Autodesk Inventor part; units mm, degrees
(part 5 of 7)
  line L3426 (-193.7386, -22.8386) -> (-193.9136, -22.7248)
  line L3427 (-193.9136, -22.7248) -> (-194.0733, -22.5914)
  line L3428 (-194.0733, -22.5914) -> (-194.216, -22.4401)
  line L3429 (-194.216, -22.4401) -> (-194.3401, -22.2722)
  line L3430 (-194.3401, -22.2722) -> (-194.4984, -22.0026)
  line L3431 (-194.4984, -22.0026) -> (-194.6175, -21.7136)
  line L3432 (-194.6175, -21.7136) -> (-194.7614, -21.1878)
  line L3433 (-194.7614, -21.1878) -> (-194.8323, -20.6472)
  line L3434 (-194.8323, -20.6472) -> (-194.8479, -20.2469)
  line L3435 (-194.8479, -20.2469) -> (-194.8362, -19.8464)
  line L3436 (-194.8323, 26.7434) -> (-194.7794, 27.1173)
  line L3437 (-194.7794, 27.1173) -> (-194.6772, 27.4752)
  line L3438 (-194.6772, 27.4752) -> (-194.5286, 27.8131)
  line L3439 (-194.5286, 27.8131) -> (-194.3367, 28.1265)
  line L3440 (-194.3367, 28.1265) -> (-194.1044, 28.4114)
  line L3441 (-194.1044, 28.4114) -> (-193.8348, 28.6634)
  line L3442 (-193.8348, 28.6634) -> (-193.5309, 28.8783)
  line L3443 (-193.5309, 28.8783) -> (-193.1956, 29.052)
  line L3444 (-193.1956, 29.052) -> (-192.8739, 29.1738)
  line L3445 (-192.8739, 29.1738) -> (-192.5434, 29.2669)
  line L3446 (-192.5434, 29.2669) -> (-192.2059, 29.3306)
  line L3447 (-192.2059, 29.3306) -> (-191.8636, 29.3645)
  line L3448 (-191.8636, 29.3645) -> (-191.5218, 29.3735)
  line L3449 (-191.5218, 29.3735) -> (-191.18, 29.3684)
  line L3450 (-191.18, 29.3684) -> (-191.18, 24.5364)
  line L3451 (-191.18, 24.5364) -> (-190.8858, 24.5593)
  line L3452 (-190.8858, 24.5593) -> (-190.5962, 24.6116)
  line L3453 (-190.5962, 24.6116) -> (-190.3134, 24.6926)
  line L3454 (-190.3134, 24.6926) -> (-190.0394, 24.802)
  line L3455 (-190.0394, 24.802) -> (-189.8038, 24.9316)
  line L3456 (-189.8038, 24.9316) -> (-189.5931, 25.0917)
  line L3457 (-189.5931, 25.0917) -> (-189.4096, 25.2786)
  line L3458 (-189.4096, 25.2786) -> (-189.2554, 25.489)
  line L3459 (-189.2554, 25.489) -> (-189.1329, 25.7192)
  line L3460 (-189.1329, 25.7192) -> (-189.0441, 25.9657)
  line L3461 (-189.0441, 25.9657) -> (-188.9913, 26.2249)
  line L3462 (-188.9913, 26.2249) -> (-188.9769, 26.4934)
  line L3463 (-188.9769, 26.4934) -> (-188.9951, 26.7775)
  line L3464 (-188.9951, 26.7775) -> (-189.055, 27.0559)
  line L3465 (-189.055, 27.0559) -> (-189.1523, 27.3014)
  line L3466 (-189.1523, 27.3014) -> (-189.2933, 27.5246)
  line L3467 (-189.2933, 27.5246) -> (-189.4825, 27.7331)
  line L3468 (-189.4825, 27.7331) -> (-189.7034, 27.9075)
  line L3469 (-189.7034, 27.9075) -> (-189.9949, 28.0747)
  line L3470 (-189.9949, 28.0747) -> (-190.305, 28.2043)
  line L3471 (-190.305, 28.2043) -> (-190.1644, 29.3411)
  line L3472 (-190.1644, 29.3411) -> (-189.8262, 29.2325)
  line L3473 (-189.8262, 29.2325) -> (-189.5048, 29.0844)
  line L3474 (-189.5048, 29.0844) -> (-189.2036, 28.8986)
  line L3475 (-189.2036, 28.8986) -> (-188.9261, 28.677)
  line L3476 (-188.9261, 28.677) -> (-188.6508, 28.3766)
  line L3477 (-188.6508, 28.3766) -> (-188.4271, 28.0391)
  line L3478 (-188.4271, 28.0391) -> (-188.2585, 27.6709)
  line L3479 (-188.2585, 27.6709) -> (-188.1487, 27.2786)
  line L3480 (-188.1487, 27.2786) -> (-188.0874, 26.8353)
  line L3481 (-188.0874, 26.8353) -> (-188.0749, 26.3893)
  line L3482 (-188.0749, 26.3893) -> (-188.111, 25.9446)
  line L3483 (-188.111, 25.9446) -> (-188.1956, 25.5051)
  line L3484 (-188.1956, 25.5051) -> (-188.3053, 25.1774)
  line L3485 (-188.3053, 25.1774) -> (-188.4537, 24.8698)
  line L3486 (-188.4537, 24.8698) -> (-188.6379, 24.5853)
  line L3487 (-188.6379, 24.5853) -> (-188.8553, 24.3267)
  line L3488 (-188.8553, 24.3267) -> (-189.103, 24.0971)
  line L3489 (-189.103, 24.0971) -> (-189.3783, 23.8992)
  line L3490 (-189.3783, 23.8992) -> (-189.6783, 23.7361)
  line L3491 (-189.6783, 23.7361) -> (-190.0003, 23.6106)
  line L3492 (-190.0003, 23.6106) -> (-190.3447, 23.5156)
  line L3493 (-190.3447, 23.5156) -> (-190.6949, 23.4486)
  line L3494 (-190.6949, 23.4486) -> (-191.0495, 23.4099)
  line L3495 (-191.0495, 23.4099) -> (-191.4065, 23.3996)
  line L3496 (-191.4065, 23.3996) -> (-191.7751, 23.4106)
  line L3497 (-191.7751, 23.4106) -> (-192.1412, 23.4495)
  line L3498 (-192.1412, 23.4495) -> (-192.5033, 23.5163)
  line L3499 (-192.5033, 23.5163) -> (-192.8597, 23.6106)
  line L3500 (-192.8597, 23.6106) -> (-193.1496, 23.7194)
  line L3501 (-193.1496, 23.7194) -> (-193.4237, 23.8577)
  line L3502 (-193.4237, 23.8577) -> (-193.6798, 24.0239)
  line L3503 (-193.6798, 24.0239) -> (-193.9159, 24.216)
  line L3504 (-193.9159, 24.216) -> (-194.1301, 24.4323)
  line L3505 (-194.1301, 24.4323) -> (-194.3205, 24.671)
  line L3506 (-194.3205, 24.671) -> (-194.4849, 24.9302)
  line L3507 (-194.4849, 24.9302) -> (-194.6214, 25.2082)
  line L3508 (-194.6214, 25.2082) -> (-194.7415, 25.5808)
  line L3509 (-194.7415, 25.5808) -> (-194.8171, 25.9634)
  line L3510 (-194.8171, 25.9634) -> (-194.8476, 26.3523)
  line L3511 (-194.8476, 26.3523) -> (-194.8323, 26.7434)
  line L3512 (-194.6995, -35.8152) -> (-194.6995, -34.7097)
  line L3513 (-194.6995, -34.7097) -> (-193.8479, -34.7097)
  line L3514 (-193.8479, -34.7097) -> (-193.8479, -35.8152)
  line L3515 (-193.8479, -35.8152) -> (-190.055, -35.8152)
  line L3516 (-190.055, -35.8152) -> (-189.7519, -35.8093)
  line L3517 (-189.7519, -35.8093) -> (-189.4534, -35.7566)
  line L3518 (-189.4534, -35.7566) -> (-189.3323, -35.6785)
  line L3519 (-189.3323, -35.6785) -> (-189.2386, -35.5691)
  line L3520 (-189.2386, -35.5691) -> (-189.1744, -35.3848)
  line L3521 (-189.1744, -35.3848) -> (-189.1604, -35.1902)
  line L3522 (-189.1604, -35.1902) -> (-189.1708, -34.949)
  line L3523 (-189.1708, -34.949) -> (-189.2034, -34.7097)
  line L3524 (-189.2034, -34.7097) -> (-188.2308, -34.5496)
  line L3525 (-188.2308, -34.5496) -> (-188.1681, -34.8873)
  line L3526 (-188.1681, -34.8873) -> (-188.1387, -35.2287)
  line L3527 (-188.1387, -35.2287) -> (-188.1426, -35.5714)
  line L3528 (-188.1426, -35.5714) -> (-188.18, -35.9128)
  line L3529 (-188.18, -35.9128) -> (-188.2439, -36.1415)
  line L3530 (-188.2439, -36.1415) -> (-188.3496, -36.3516)
  line L3531 (-188.3496, -36.3516) -> (-188.4935, -36.5377)
  line L3532 (-188.4935, -36.5377) -> (-188.6722, -36.6941)
  line L3533 (-188.6722, -36.6941) -> (-188.8197, -36.7661)
  line L3534 (-188.8197, -36.7661) -> (-188.9742, -36.8204)
  line L3535 (-188.9742, -36.8204) -> (-189.1338, -36.8564)
  line L3536 (-189.1338, -36.8564) -> (-189.2972, -36.8738)
  line L3537 (-189.2972, -36.8738) -> (-189.707, -36.8995)
  line L3538 (-189.707, -36.8995) -> (-190.1175, -36.9089)
  line L3539 (-190.1175, -36.9089) -> (-193.8479, -36.9089)
  line L3540 (-193.8479, -36.9089) -> (-193.8479, -37.7136)
  line L3541 (-193.8479, -37.7136) -> (-194.6995, -37.7136)
  line L3542 (-194.6995, -37.7136) -> (-194.6995, -36.9089)
  line L3543 (-194.6995, -36.9089) -> (-196.305, -36.9089)
  line L3544 (-196.305, -36.9089) -> (-196.9651, -35.8152)
  line L3545 (-196.9651, -35.8152) -> (-194.6995, -35.8152)
  line L3546 (-194.8401, 20.2825) -> (-194.8127, 20.5351)
  line L3547 (-194.8127, 20.5351) -> (-194.7541, 20.7814)
  line L3548 (-194.7541, 20.7814) -> (-194.6653, 21.0184)
  line L3549 (-194.6653, 21.0184) -> (-194.5472, 21.2434)
  line L3550 (-194.5472, 21.2434) -> (-194.3696, 21.4735)
  line L3551 (-194.3696, 21.4735) -> (-194.1547, 21.6657)
  line L3552 (-194.1547, 21.6657) -> (-193.9086, 21.8157)
  line L3553 (-193.9086, 21.8157) -> (-193.637, 21.9192)
  line L3554 (-193.637, 21.9192) -> (-193.3991, 21.9795)
  line L3555 (-193.3991, 21.9795) -> (-193.1576, 22.0212)
  line L3556 (-193.1576, 22.0212) -> (-192.9136, 22.0441)
  line L3557 (-192.9136, 22.0441) -> (-192.6683, 22.0481)
  line L3558 (-192.6683, 22.0481) -> (-188.219, 22.0481)
  line L3559 (-188.219, 22.0481) -> (-188.219, 20.9583)
  line L3560 (-188.219, 20.9583) -> (-192.3011, 20.9583)
  line L3561 (-192.3011, 20.9583) -> (-192.6934, 20.9484)
  line L3562 (-192.6934, 20.9484) -> (-193.0823, 20.8958)
  line L3563 (-193.0823, 20.8958) -> (-193.274, 20.8411)
  line L3564 (-193.274, 20.8411) -> (-193.4477, 20.748)
  line L3565 (-193.4477, 20.748) -> (-193.598, 20.6205)
  line L3566 (-193.598, 20.6205) -> (-193.719, 20.4622)
  line L3567 (-193.719, 20.4622) -> (-193.8114, 20.2685)
  line L3568 (-193.8114, 20.2685) -> (-193.8707, 20.0638)
  line L3569 (-193.8707, 20.0638) -> (-193.8962, 19.8523)
  line L3570 (-193.8962, 19.8523) -> (-193.887, 19.6379)
  line L3571 (-193.887, 19.6379) -> (-193.8564, 19.4131)
  line L3572 (-193.8564, 19.4131) -> (-193.7925, 19.1996)
  line L3573 (-193.7925, 19.1996) -> (-193.6978, 19.0006)
  line L3574 (-193.6978, 19.0006) -> (-193.5748, 18.819)
  line L3575 (-193.5748, 18.819) -> (-193.4259, 18.658)
  line L3576 (-193.4259, 18.658) -> (-193.2534, 18.5207)
  line L3577 (-193.2534, 18.5207) -> (-193.06, 18.4101)
  line L3578 (-193.06, 18.4101) -> (-192.8479, 18.3293)
  line L3579 (-192.8479, 18.3293) -> (-192.4207, 18.2395)
  line L3580 (-192.4207, 18.2395) -> (-191.9847, 18.2161)
  line L3581 (-191.9847, 18.2161) -> (-188.219, 18.2161)
  line L3582 (-188.219, 18.2161) -> (-188.219, 17.1184)
  line L3583 (-188.219, 17.1184) -> (-192.43, 17.1184)
  line L3584 (-192.43, 17.1184) -> (-192.7524, 17.1051)
  line L3585 (-192.7524, 17.1051) -> (-193.0706, 17.052)
  line L3586 (-193.0706, 17.052) -> (-193.3245, 16.9661)
  line L3587 (-193.3245, 16.9661) -> (-193.5276, 16.8489)
  line L3588 (-193.5276, 16.8489) -> (-193.658, 16.7293)
  line L3589 (-193.658, 16.7293) -> (-193.7605, 16.5873)
  line L3590 (-193.7605, 16.5873) -> (-193.8326, 16.4277)
  line L3591 (-193.8326, 16.4277) -> (-193.8714, 16.2551)
  line L3592 (-193.8714, 16.2551) -> (-193.8959, 15.9585)
  line L3593 (-193.8959, 15.9585) -> (-193.8667, 15.6647)
  line L3594 (-193.8667, 15.6647) -> (-193.7851, 15.381)
  line L3595 (-193.7851, 15.381) -> (-193.6526, 15.1145)
  line L3596 (-193.6526, 15.1145) -> (-193.5526, 14.9735)
  line L3597 (-193.5526, 14.9735) -> (-193.4355, 14.8474)
  line L3598 (-193.4355, 14.8474) -> (-193.3029, 14.7376)
  line L3599 (-193.3029, 14.7376) -> (-193.1565, 14.6458)
  line L3600 (-193.1565, 14.6458) -> (-192.9228, 14.5385)
  line L3601 (-192.9228, 14.5385) -> (-192.6761, 14.4661)
  line L3602 (-192.6761, 14.4661) -> (-192.1319, 14.3864)
  line L3603 (-192.1319, 14.3864) -> (-191.5823, 14.3645)
  line L3604 (-191.5823, 14.3645) -> (-188.219, 14.3645)
  line L3605 (-188.219, 14.3645) -> (-188.219, 13.2668)
  line L3606 (-188.219, 13.2668) -> (-194.6995, 13.2668)
  line L3607 (-194.6995, 13.2668) -> (-194.6995, 14.2512)
  line L3608 (-194.6995, 14.2512) -> (-193.7933, 14.2512)
  line L3609 (-193.7933, 14.2512) -> (-194.0001, 14.3989)
  line L3610 (-194.0001, 14.3989) -> (-194.1874, 14.5672)
  line L3611 (-194.1874, 14.5672) -> (-194.3537, 14.7542)
  line L3612 (-194.3537, 14.7542) -> (-194.498, 14.9579)
  line L3613 (-194.498, 14.9579) -> (-194.6188, 15.1763)
  line L3614 (-194.6188, 15.1763) -> (-194.715, 15.4074)
  line L3615 (-194.715, 15.4074) -> (-194.7853, 15.6492)
  line L3616 (-194.7853, 15.6492) -> (-194.8284, 15.8997)
  line L3617 (-194.8284, 15.8997) -> (-194.8467, 16.143)
  line L3618 (-194.8467, 16.143) -> (-194.8436, 16.3864)
  line L3619 (-194.8436, 16.3864) -> (-194.8193, 16.6287)
  line L3620 (-194.8193, 16.6287) -> (-194.7737, 16.8684)
  line L3621 (-194.7737, 16.8684) -> (-194.68, 17.1497)
  line L3622 (-194.68, 17.1497) -> (-194.588, 17.3313)
  line L3623 (-194.588, 17.3313) -> (-194.4751, 17.4999)
  line L3624 (-194.4751, 17.4999) -> (-194.3425, 17.6534)
  line L3625 (-194.3425, 17.6534) -> (-194.1917, 17.7903)
  line L3626 (-194.1917, 17.7903) -> (-193.9617, 17.9366)
  line L3627 (-193.9617, 17.9366) -> (-193.7112, 18.0442)
  line L3628 (-193.7112, 18.0442) -> (-193.9614, 18.2279)
  line L3629 (-193.9614, 18.2279) -> (-194.1882, 18.4384)
  line L3630 (-194.1882, 18.4384) -> (-194.3894, 18.6735)
  line L3631 (-194.3894, 18.6735) -> (-194.5628, 18.9309)
  line L3632 (-194.5628, 18.9309) -> (-194.6614, 19.1236)
  line L3633 (-194.6614, 19.1236) -> (-194.739, 19.325)
  line L3634 (-194.739, 19.325) -> (-194.7948, 19.5335)
  line L3635 (-194.7948, 19.5335) -> (-194.8284, 19.7473)
  line L3636 (-194.8284, 19.7473) -> (-194.8474, 20.0146)
  line L3637 (-194.8474, 20.0146) -> (-194.8401, 20.2825)
  line L3638 (-188.219, 11.6223) -> (-188.219, 10.5247)
  line L3639 (-188.219, 10.5247) -> (-194.6995, 10.5247)
  line L3640 (-194.6995, 10.5247) -> (-194.6995, 11.6223)
  line L3641 (-194.6995, 11.6223) -> (-188.219, 11.6223)
  line L3642 (-197.1644, -2.0066) -> (-197.1365, -1.3334)
  line L3643 (-197.1365, -1.3334) -> (-197.0394, -0.6667)
  line L3644 (-197.0394, -0.6667) -> (-196.9661, -0.397)
  line L3645 (-196.9661, -0.397) -> (-196.8703, -0.1349)
  line L3646 (-196.8703, -0.1349) -> (-196.7526, 0.1181)
  line L3647 (-196.7526, 0.1181) -> (-196.6136, 0.3606)
  line L3648 (-196.6136, 0.3606) -> (-196.3987, 0.6458)
  line L3649 (-196.3987, 0.6458) -> (-196.0784, 0.9778)
  line L3650 (-196.0784, 0.9778) -> (-195.7151, 1.2629)
  line L3651 (-195.7151, 1.2629) -> (-195.3128, 1.5051)
  line L3652 (-195.3128, 1.5051) -> (-194.8675, 1.7043)
  line L3653 (-194.8675, 1.7043) -> (-194.387, 1.8567)
  line L3654 (-194.387, 1.8567) -> (-193.8596, 1.968)
  line L3655 (-193.8596, 1.968) -> (-193.3245, 2.0325)
  line L3656 (-193.3245, 2.0325) -> (-192.9384, 2.0538)
  line L3657 (-192.9384, 2.0538) -> (-192.552, 2.0544)
  line L3658 (-192.552, 2.0544) -> (-192.1661, 2.0342)
  line L3659 (-192.1661, 2.0342) -> (-191.7815, 1.9934)
  line L3660 (-191.7815, 1.9934) -> (-191.2923, 1.9097)
  line L3661 (-191.2923, 1.9097) -> (-190.8145, 1.7795)
  line L3662 (-190.8145, 1.7795) -> (-190.3515, 1.6039)
  line L3663 (-190.3515, 1.6039) -> (-189.9065, 1.384)
  line L3664 (-189.9065, 1.384) -> (-189.5949, 1.1825)
  line L3665 (-189.5949, 1.1825) -> (-189.3083, 0.9484)
  line L3666 (-189.3083, 0.9484) -> (-189.0494, 0.6841)
  line L3667 (-189.0494, 0.6841) -> (-188.8206, 0.3918)
  line L3668 (-188.8206, 0.3918) -> (-188.6377, 0.0648)
  line L3669 (-188.6377, 0.0648) -> (-188.4901, -0.2785)
  line L3670 (-188.4901, -0.2785) -> (-188.3788, -0.6353)
  line L3671 (-188.3788, -0.6353) -> (-188.305, -1.0027)
  line L3672 (-188.305, -1.0027) -> (-188.2376, -1.5574)
  line L3673 (-188.2376, -1.5574) -> (-188.219, -2.116)
  line L3674 (-188.219, -2.116) -> (-188.219, -5.3425)
  line L3675 (-188.219, -5.3425) -> (-197.1683, -5.3425)
  line L3676 (-197.1683, -5.3425) -> (-197.1683, -2.2605)
  line L3677 (-197.1683, -2.2605) -> (-197.1644, -2.0066)
  line L3678 (-194.8362, -12.6433) -> (-194.7875, -12.3186)
  line L3679 (-194.7875, -12.3186) -> (-194.6967, -12.0045)
  line L3680 (-194.6967, -12.0045) -> (-194.5653, -11.7052)
  line L3681 (-194.5653, -11.7052) -> (-194.3948, -11.4246)
  line L3682 (-194.3948, -11.4246) -> (-194.2515, -11.2623)
  line L3683 (-194.2515, -11.2623) -> (-194.0882, -11.1217)
  line L3684 (-194.0882, -11.1217) -> (-193.9073, -11.0046)
  line L3685 (-193.9073, -11.0046) -> (-193.7112, -10.9128)
  line L3686 (-193.7112, -10.9128) -> (-193.504, -10.8357)
  line L3687 (-193.504, -10.8357) -> (-193.2906, -10.7799)
  line L3688 (-193.2906, -10.7799) -> (-193.0726, -10.7456)
  line L3689 (-193.0726, -10.7456) -> (-192.8519, -10.7332)
  line L3690 (-192.8519, -10.7332) -> (-192.5278, -10.7206)
  line L3691 (-192.5278, -10.7206) -> (-192.2034, -10.7175)
  line L3692 (-192.2034, -10.7175) -> (-188.219, -10.7175)
  line L3693 (-188.219, -10.7175) -> (-188.219, -11.8152)
  line L3694 (-188.219, -11.8152) -> (-192.1604, -11.8152)
  line L3695 (-192.1604, -11.8152) -> (-192.5707, -11.8269)
  line L3696 (-192.5707, -11.8269) -> (-192.9769, -11.8855)
  line L3697 (-192.9769, -11.8855) -> (-193.2395, -11.9747)
  line L3698 (-193.2395, -11.9747) -> (-193.4685, -12.124)
  line L3699 (-193.4685, -12.124) -> (-193.6538, -12.3249)
  line L3700 (-193.6538, -12.3249) -> (-193.7854, -12.5691)
  line L3701 (-193.7854, -12.5691) -> (-193.8689, -12.8607)
  line L3702 (-193.8689, -12.8607) -> (-193.8948, -13.1628)
  line L3703 (-193.8948, -13.1628) -> (-193.8675, -13.5027)
  line L3704 (-193.8675, -13.5027) -> (-193.7854, -13.8191)
  line L3705 (-193.7854, -13.8191) -> (-193.6448, -14.1082)
  line L3706 (-193.6448, -14.1082) -> (-193.4495, -14.3738)
  line L3707 (-193.4495, -14.3738) -> (-193.3097, -14.5026)
  line L3708 (-193.3097, -14.5026) -> (-193.1541, -14.6103)
  line L3709 (-193.1541, -14.6103) -> (-192.9851, -14.6955)
  line L3710 (-192.9851, -14.6955) -> (-192.805, -14.7566)
  line L3711 (-192.805, -14.7566) -> (-192.5474, -14.8178)
  line L3712 (-192.5474, -14.8178) -> (-192.2863, -14.8598)
  line L3713 (-192.2863, -14.8598) -> (-192.0229, -14.8824)
  line L3714 (-192.0229, -14.8824) -> (-191.7581, -14.8855)
  line L3715 (-191.7581, -14.8855) -> (-188.219, -14.8855)
  line L3716 (-188.219, -14.8855) -> (-188.219, -15.9832)
  line L3717 (-188.219, -15.9832) -> (-194.6995, -15.9832)
  line L3718 (-194.6995, -15.9832) -> (-194.6995, -14.9949)
  line L3719 (-194.6995, -14.9949) -> (-193.7776, -14.9949)
  line L3720 (-193.7776, -14.9949) -> (-194.0195, -14.816)
  line L3721 (-194.0195, -14.816) -> (-194.2358, -14.6087)
  line L3722 (-194.2358, -14.6087) -> (-194.4242, -14.3758)
  line L3723 (-194.4242, -14.3758) -> (-194.5823, -14.1199)
  line L3724 (-194.5823, -14.1199) -> (-194.702, -13.8366)
  line L3725 (-194.702, -13.8366) -> (-194.7866, -13.5421)
  line L3726 (-194.7866, -13.5421) -> (-194.8355, -13.2396)
  line L3727 (-194.8355, -13.2396) -> (-194.8479, -12.9324)
  line L3728 (-194.8479, -12.9324) -> (-194.8362, -12.6433)
  line L3729 (-197.3128, -24.3152) -> (-197.2749, -23.919)
  line L3730 (-197.2749, -23.919) -> (-197.2112, -23.5261)
  line L3731 (-197.2112, -23.5261) -> (-196.2503, -23.6902)
  line L3732 (-196.2503, -23.6902) -> (-196.2963, -24.013)
  line L3733 (-196.2963, -24.013) -> (-196.3128, -24.3386)
  line L3734 (-196.3128, -24.3386) -> (-196.2993, -24.5533)
  line L3735 (-196.2993, -24.5533) -> (-196.2581, -24.7644)
  line L3736 (-196.2581, -24.7644) -> (-196.1968, -24.9157)
  line L3737 (-196.1968, -24.9157) -> (-196.0979, -25.0457)
  line L3738 (-196.0979, -25.0457) -> (-195.969, -25.1355)
  line L3739 (-195.969, -25.1355) -> (-195.7748, -25.207)
  line L3740 (-195.7748, -25.207) -> (-195.5706, -25.241)
  line L3741 (-195.5706, -25.241) -> (-195.1352, -25.2563)
  line L3742 (-195.1352, -25.2563) -> (-194.6995, -25.2527)
  line L3743 (-194.6995, -25.2527) -> (-194.6995, -23.991)
  line L3744 (-194.6995, -23.991) -> (-193.8479, -23.991)
  line L3745 (-193.8479, -23.991) -> (-193.8479, -25.2527)
  line L3746 (-193.8479, -25.2527) -> (-188.219, -25.2527)
  line L3747 (-188.219, -25.2527) -> (-188.219, -26.3464)
  line L3748 (-188.219, -26.3464) -> (-193.8479, -26.3464)
  line L3749 (-193.8479, -26.3464) -> (-193.8479, -27.3152)
  line L3750 (-193.8479, -27.3152) -> (-194.6995, -27.3152)
  line L3751 (-194.6995, -27.3152) -> (-194.6995, -26.3464)
  line L3752 (-194.6995, -26.3464) -> (-195.1976, -26.3489)
  line L3753 (-195.1976, -26.3489) -> (-195.6956, -26.3386)
  line L3754 (-195.6956, -26.3386) -> (-196.0317, -26.3088)
  line L3755 (-196.0317, -26.3088) -> (-196.3597, -26.2293)
  line L3756 (-196.3597, -26.2293) -> (-196.6195, -26.1015)
  line L3757 (-196.6195, -26.1015) -> (-196.8453, -25.9252)
  line L3758 (-196.8453, -25.9252) -> (-197.0304, -25.7065)
  line L3759 (-197.0304, -25.7065) -> (-197.1683, -25.4519)
  line L3760 (-197.1683, -25.4519) -> (-197.2542, -25.1902)
  line L3761 (-197.2542, -25.1902) -> (-197.3134, -24.7547)
  line L3762 (-197.3134, -24.7547) -> (-197.3128, -24.3152)
  line L3763 (-188.219, 31.8411) -> (-188.219, 30.7434)
  line L3764 (-188.219, 30.7434) -> (-197.1683, 30.7434)
  line L3765 (-197.1683, 30.7434) -> (-197.1683, 31.8411)
  line L3766 (-197.1683, 31.8411) -> (-188.219, 31.8411)
  line L3767 (-191.4104, -19.0027) -> (-191.1986, -19.8133)
  line L3768 (-191.1986, -19.8133) -> (-191.0589, -20.6394)
  line L3769 (-191.0589, -20.6394) -> (-190.9765, -21.1247)
  line L3770 (-190.9765, -21.1247) -> (-190.8362, -21.5964)
  line L3771 (-190.8362, -21.5964) -> (-190.6926, -21.84)
  line L3772 (-190.6926, -21.84) -> (-190.4877, -22.0259)
  line L3773 (-190.4877, -22.0259) -> (-190.2373, -22.1435)
  line L3774 (-190.2373, -22.1435) -> (-189.9573, -22.1824)
  line L3775 (-189.9573, -22.1824) -> (-189.7515, -22.1639)
  line L3776 (-189.7515, -22.1639) -> (-189.555, -22.1003)
  line L3777 (-189.555, -22.1003) -> (-189.4166, -22.0194)
  line L3778 (-189.4166, -22.0194) -> (-189.2929, -21.9189)
  line L3779 (-189.2929, -21.9189) -> (-189.186, -21.8007)
  line L3780 (-189.186, -21.8007) -> (-189.0979, -21.6668)
  line L3781 (-189.0979, -21.6668) -> (-189.0047, -21.4288)
  line L3782 (-189.0047, -21.4288) -> (-188.9534, -21.1785)
  line L3783 (-188.9534, -21.1785) -> (-188.9323, -20.8798)
  line L3784 (-188.9323, -20.8798) -> (-188.9483, -20.582)
  line L3785 (-188.9483, -20.582) -> (-189.0011, -20.2885)
  line L3786 (-189.0011, -20.2885) -> (-189.0901, -20.0027)
  line L3787 (-189.0901, -20.0027) -> (-189.1751, -19.8148)
  line L3788 (-189.1751, -19.8148) -> (-189.2789, -19.6374)
  line L3789 (-189.2789, -19.6374) -> (-189.4007, -19.4716)
  line L3790 (-189.4007, -19.4716) -> (-189.5394, -19.3191)
  line L3791 (-189.5394, -19.3191) -> (-189.7431, -19.1546)
  line L3792 (-189.7431, -19.1546) -> (-189.969, -19.0222)
  line L3793 (-189.969, -19.0222) -> (-190.3406, -18.9061)
  line L3794 (-190.3406, -18.9061) -> (-190.7269, -18.8582)
  line L3795 (-190.7269, -18.8582) -> (-191.0998, -18.8459)
  line L3796 (-191.0998, -18.8459) -> (-191.4729, -18.8464)
  line L3797 (-191.4729, -18.8464) -> (-191.4104, -19.0027)
  line L3798 (-196.1097, -4.1589) -> (-189.2737, -4.1589)
  line L3799 (-189.2737, -4.1589) -> (-189.2737, -2.2488)
  line L3800 (-189.2737, -2.2488) -> (-189.293, -1.6898)
  line L3801 (-189.293, -1.6898) -> (-189.3675, -1.1355)
  line L3802 (-189.3675, -1.1355) -> (-189.4284, -0.8919)
  line L3803 (-189.4284, -0.8919) -> (-189.515, -0.657)
  line L3804 (-189.515, -0.657) -> (-189.6265, -0.4328)
  line L3805 (-189.6265, -0.4328) -> (-189.762, -0.2214)
  line L3806 (-189.762, -0.2214) -> (-189.9026, -0.0574)
  line L3807 (-189.9026, -0.0574) -> (-190.0834, 0.101)
  line L3808 (-190.0834, 0.101) -> (-190.2773, 0.2422)
  line L3809 (-190.2773, 0.2422) -> (-190.483, 0.3655)
  line L3810 (-190.483, 0.3655) -> (-190.6995, 0.47)
  line L3811 (-190.6995, 0.47) -> (-190.9715, 0.5747)
  line L3812 (-190.9715, 0.5747) -> (-191.2496, 0.6606)
  line L3813 (-191.2496, 0.6606) -> (-191.533, 0.7273)
  line L3814 (-191.533, 0.7273) -> (-191.8206, 0.7747)
  line L3815 (-191.8206, 0.7747) -> (-192.2955, 0.8194)
  line L3816 (-192.2955, 0.8194) -> (-192.7719, 0.8336)
  line L3817 (-192.7719, 0.8336) -> (-193.2482, 0.8174)
  line L3818 (-193.2482, 0.8174) -> (-193.7229, 0.7708)
  line L3819 (-193.7229, 0.7708) -> (-193.9794, 0.726)
  line L3820 (-193.9794, 0.726) -> (-194.2316, 0.6627)
  line L3821 (-194.2316, 0.6627) -> (-194.4785, 0.5812)
  line L3822 (-194.4785, 0.5812) -> (-194.719, 0.4817)
  line L3823 (-194.719, 0.4817) -> (-195.0263, 0.3093)
  line L3824 (-195.0263, 0.3093) -> (-195.3063, 0.0981)
  line L3825 (-195.3063, 0.0981) -> (-195.5554, -0.1489)
  line L3826 (-195.5554, -0.1489) -> (-195.7698, -0.4285)
  line L3827 (-195.7698, -0.4285) -> (-195.8835, -0.6501)
  line L3828 (-195.8835, -0.6501) -> (-195.9713, -0.8824)
  line L3829 (-195.9713, -0.8824) -> (-196.0326, -1.1231)
  line L3830 (-196.0326, -1.1231) -> (-196.0667, -1.3699)
  line L3831 (-196.0667, -1.3699) -> (-196.0928, -1.6957)
  line L3832 (-196.0928, -1.6957) -> (-196.1097, -2.0222)
  line L3833 (-196.1097, -2.0222) -> (-196.1097, -4.1589)
  line L3834 (-193.9378, 6.0051) -> (-193.8934, 5.7383)
  line L3835 (-193.8934, 5.7383) -> (-193.811, 5.4854)
  line L3836 (-193.811, 5.4854) -> (-193.6932, 5.2501)
  line L3837 (-193.6932, 5.2501) -> (-193.543, 5.0355)
  line L3838 (-193.543, 5.0355) -> (-193.3629, 4.8453)
  line L3839 (-193.3629, 4.8453) -> (-193.1559, 4.6827)
  line L3840 (-193.1559, 4.6827) -> (-192.9247, 4.5513)
  line L3841 (-192.9247, 4.5513) -> (-192.6722, 4.4543)
  line L3842 (-192.6722, 4.4543) -> (-192.3803, 4.3834)
  line L3843 (-192.3803, 4.3834) -> (-192.0823, 4.345)
  line L3844 (-192.0823, 4.345) -> (-192.0823, 7.9661)
  line L3845 (-192.0823, 7.9661) -> (-192.4436, 7.9157)
  line L3846 (-192.4436, 7.9157) -> (-192.7972, 7.8254)
  line L3847 (-192.7972, 7.8254) -> (-193.0784, 7.7043)
  line L3848 (-193.0784, 7.7043) -> (-193.3089, 7.552)
  line L3849 (-193.3089, 7.552) -> (-193.5836, 7.2736)
  line L3850 (-193.5836, 7.2736) -> (-193.7856, 6.9443)
  line L3851 (-193.7856, 6.9443) -> (-193.9085, 6.5781)
  line L3852 (-193.9085, 6.5781) -> (-193.9456, 6.1887)
  line L3853 (-193.9456, 6.1887) -> (-193.9378, 6.0051)
  line L3854 (-193.9378, -31.1199) -> (-193.8934, -31.3867)
  line L3855 (-193.8934, -31.3867) -> (-193.811, -31.6396)
  line L3856 (-193.811, -31.6396) -> (-193.6932, -31.8749)
  line L3857 (-193.6932, -31.8749) -> (-193.543, -32.0895)
  line L3858 (-193.543, -32.0895) -> (-193.3629, -32.2797)
  line L3859 (-193.3629, -32.2797) -> (-193.1559, -32.4423)
  line L3860 (-193.1559, -32.4423) -> (-192.9247, -32.5737)
  line L3861 (-192.9247, -32.5737) -> (-192.6722, -32.6707)
  line L3862 (-192.6722, -32.6707) -> (-192.3803, -32.7416)
  line L3863 (-192.3803, -32.7416) -> (-192.0823, -32.78)
  line L3864 (-192.0823, -32.78) -> (-192.0823, -29.1589)
  line L3865 (-192.0823, -29.1589) -> (-192.4436, -29.2093)
  line L3866 (-192.4436, -29.2093) -> (-192.7972, -29.2996)
  line L3867 (-192.7972, -29.2996) -> (-193.0784, -29.4207)
  line L3868 (-193.0784, -29.4207) -> (-193.3089, -29.573)
  line L3869 (-193.3089, -29.573) -> (-193.5836, -29.8514)
  line L3870 (-193.5836, -29.8514) -> (-193.7856, -30.1807)
  line L3871 (-193.7856, -30.1807) -> (-193.9085, -30.5469)
  line L3872 (-193.9085, -30.5469) -> (-193.9456, -30.9363)
  line L3873 (-193.9456, -30.9363) -> (-193.9378, -31.1199)
  line L3874 (-193.9378, 26.2551) -> (-193.8934, 25.9883)
  line L3875 (-193.8934, 25.9883) -> (-193.811, 25.7354)
  line L3876 (-193.811, 25.7354) -> (-193.6932, 25.5001)
  line L3877 (-193.6932, 25.5001) -> (-193.543, 25.2855)
  line L3878 (-193.543, 25.2855) -> (-193.3629, 25.0953)
  line L3879 (-193.3629, 25.0953) -> (-193.1559, 24.9327)
  line L3880 (-193.1559, 24.9327) -> (-192.9247, 24.8013)
  line L3881 (-192.9247, 24.8013) -> (-192.6722, 24.7043)
  line L3882 (-192.6722, 24.7043) -> (-192.3803, 24.6334)
  line L3883 (-192.3803, 24.6334) -> (-192.0823, 24.595)
  line L3884 (-192.0823, 24.595) -> (-192.0823, 28.2161)
  line L3885 (-192.0823, 28.2161) -> (-192.4436, 28.1657)
  line L3886 (-192.4436, 28.1657) -> (-192.7972, 28.0754)
  line L3887 (-192.7972, 28.0754) -> (-193.0784, 27.9543)
  line L3888 (-193.0784, 27.9543) -> (-193.3089, 27.802)
  line L3889 (-193.3089, 27.802) -> (-193.5836, 27.5236)
  line L3890 (-193.5836, 27.5236) -> (-193.7856, 27.1944)
  line L3891 (-193.7856, 27.1944) -> (-193.9085, 26.8281)
  line L3892 (-193.9085, 26.8281) -> (-193.9456, 26.4387)
  line L3893 (-193.9456, 26.4387) -> (-193.9378, 26.2551)
  line L3894 (-195.9026, 11.6223) -> (-195.9026, 10.5247)
  line L3895 (-195.9026, 10.5247) -> (-197.1683, 10.5247)
  line L3896 (-197.1683, 10.5247) -> (-197.1683, 11.6223)
  line L3897 (-197.1683, 11.6223) -> (-195.9026, 11.6223)
  line L3898 (-227.0771, -10.9382) -> (-227.0218, -10.5293)
  line L3899 (-227.0218, -10.5293) -> (-226.9252, -10.1293)
  line L3900 (-226.9252, -10.1293) -> (-226.7884, -9.7411)
  line L3901 (-226.7884, -9.7411) -> (-226.6123, -9.3679)
  line L3902 (-226.6123, -9.3679) -> (-226.328, -8.9335)
  line L3903 (-226.328, -8.9335) -> (-225.9905, -8.542)
  line L3904 (-225.9905, -8.542) -> (-225.6045, -8.1982)
  line L3905 (-225.6045, -8.1982) -> (-225.1748, -7.907)
  line L3906 (-225.1748, -7.907) -> (-224.8741, -7.749)
  line L3907 (-224.8741, -7.749) -> (-224.5626, -7.6146)
  line L3908 (-224.5626, -7.6146) -> (-224.2418, -7.5043)
  line L3909 (-224.2418, -7.5043) -> (-223.9131, -7.4187)
  line L3910 (-223.9131, -7.4187) -> (-223.5313, -7.3452)
  line L3911 (-223.5313, -7.3452) -> (-223.1462, -7.2939)
  line L3912 (-223.1462, -7.2939) -> (-222.7588, -7.265)
  line L3913 (-222.7588, -7.265) -> (-222.3701, -7.2586)
  line L3914 (-222.3701, -7.2586) -> (-222.165, -7.2605)
  line L3915 (-222.165, -7.2605) -> (-221.9599, -7.2664)
  line L3916 (-221.9599, -7.2664) -> (-221.9599, -14.032)
  line L3917 (-221.9599, -14.032) -> (-221.6232, -14.0071)
  line L3918 (-221.6232, -14.0071) -> (-221.2899, -13.9563)
  line L3919 (-221.2899, -13.9563) -> (-220.9616, -13.8799)
  line L3920 (-220.9616, -13.8799) -> (-220.6396, -13.7781)
  line L3921 (-220.6396, -13.7781) -> (-220.3758, -13.6683)
  line L3922 (-220.3758, -13.6683) -> (-220.1251, -13.5327)
  line L3923 (-220.1251, -13.5327) -> (-219.8895, -13.3722)
  line L3924 (-219.8895, -13.3722) -> (-219.6709, -13.1882)
  line L3925 (-219.6709, -13.1882) -> (-219.4859, -12.9951)
  line L3926 (-219.4859, -12.9951) -> (-219.3237, -12.7853)
  line L3927 (-219.3237, -12.7853) -> (-219.1849, -12.5608)
  line L3928 (-219.1849, -12.5608) -> (-219.0706, -12.3238)
  line L3929 (-219.0706, -12.3238) -> (-218.9815, -12.0761)
  line L3930 (-218.9815, -12.0761) -> (-218.9184, -11.8199)
  line L3931 (-218.9184, -11.8199) -> (-218.8823, -11.5571)
  line L3932 (-218.8823, -11.5571) -> (-218.874, -11.2898)
  line L3933 (-218.874, -11.2898) -> (-218.896, -10.9049)
  line L3934 (-218.896, -10.9049) -> (-218.979, -10.5309)
  line L3935 (-218.979, -10.5309) -> (-219.1209, -10.175)
  line L3936 (-219.1209, -10.175) -> (-219.3193, -9.8445)
  line L3937 (-219.3193, -9.8445) -> (-219.4833, -9.653)
  line L3938 (-219.4833, -9.653) -> (-219.666, -9.4802)
  line L3939 (-219.666, -9.4802) -> (-219.8658, -9.3274)
  line L3940 (-219.8658, -9.3274) -> (-220.081, -9.1961)
  line L3941 (-220.081, -9.1961) -> (-220.4023, -9.0325)
  line L3942 (-220.4023, -9.0325) -> (-220.7373, -8.8992)
  line L3943 (-220.7373, -8.8992) -> (-220.542, -7.3093)
  line L3944 (-220.542, -7.3093) -> (-220.0673, -7.4583)
  line L3945 (-220.0673, -7.4583) -> (-219.6161, -7.6634)
  line L3946 (-219.6161, -7.6634) -> (-219.1933, -7.9219)
  line L3947 (-219.1933, -7.9219) -> (-218.8037, -8.2312)
  line L3948 (-218.8037, -8.2312) -> (-218.4711, -8.5837)
  line L3949 (-218.4711, -8.5837) -> (-218.1911, -8.9766)
  line L3950 (-218.1911, -8.9766) -> (-217.9675, -9.404)
  line L3951 (-217.9675, -9.404) -> (-217.8037, -9.8601)
  line L3952 (-217.8037, -9.8601) -> (-217.7168, -10.2136)
  line L3953 (-217.7168, -10.2136) -> (-217.6552, -10.572)
  line L3954 (-217.6552, -10.572) -> (-217.619, -10.9337)
  line L3955 (-217.619, -10.9337) -> (-217.6084, -11.2976)
  line L3956 (-217.6084, -11.2976) -> (-217.6271, -11.772)
  line L3957 (-217.6271, -11.772) -> (-217.6865, -12.2429)
  line L3958 (-217.6865, -12.2429) -> (-217.7819, -12.6683)
  line L3959 (-217.7819, -12.6683) -> (-217.917, -13.0828)
  line L3960 (-217.917, -13.0828) -> (-218.0427, -13.3727)
  line L3961 (-218.0427, -13.3727) -> (-218.1916, -13.6496)
  line L3962 (-218.1916, -13.6496) -> (-218.3625, -13.9122)
  line L3963 (-218.3625, -13.9122) -> (-218.5544, -14.1591)
  line L3964 (-218.5544, -14.1591) -> (-218.7663, -14.3892)
  line L3965 (-218.7663, -14.3892) -> (-218.997, -14.6011)
  line L3966 (-218.997, -14.6011) -> (-219.2455, -14.7937)
  line L3967 (-219.2455, -14.7937) -> (-219.5107, -14.9656)
  line L3968 (-219.5107, -14.9656) -> (-219.8071, -15.1226)
  line L3969 (-219.8071, -15.1226) -> (-220.1137, -15.2574)
  line L3970 (-220.1137, -15.2574) -> (-220.4294, -15.3692)
  line L3971 (-220.4294, -15.3692) -> (-220.7529, -15.4578)
  line L3972 (-220.7529, -15.4578) -> (-221.1299, -15.5304)
  line L3973 (-221.1299, -15.5304) -> (-221.5101, -15.5819)
  line L3974 (-221.5101, -15.5819) -> (-221.8925, -15.6125)
  line L3975 (-221.8925, -15.6125) -> (-222.2764, -15.6218)
  line L3976 (-222.2764, -15.6218) -> (-222.6729, -15.6137)
  line L3977 (-222.6729, -15.6137) -> (-223.068, -15.5835)
  line L3978 (-223.068, -15.5835) -> (-223.4609, -15.5315)
  line L3979 (-223.4609, -15.5315) -> (-223.8506, -15.4578)
  line L3980 (-223.8506, -15.4578) -> (-224.1851, -15.3688)
  line L3981 (-224.1851, -15.3688) -> (-224.5117, -15.2554)
  line L3982 (-224.5117, -15.2554) -> (-224.829, -15.1183)
  line L3983 (-224.829, -15.1183) -> (-225.1357, -14.9578)
  line L3984 (-225.1357, -14.9578) -> (-225.499, -14.7195)
  line L3985 (-225.499, -14.7195) -> (-225.7471, -14.5187)
  line L3986 (-225.7471, -14.5187) -> (-225.9783, -14.2994)
  line L3987 (-225.9783, -14.2994) -> (-226.1915, -14.0626)
  line L3988 (-226.1915, -14.0626) -> (-226.3857, -13.8093)
  line L3989 (-226.3857, -13.8093) -> (-226.5532, -13.5485)
  line L3990 (-226.5532, -13.5485) -> (-226.698, -13.275)
  line L3991 (-226.698, -13.275) -> (-226.8195, -12.9903)
  line L3992 (-226.8195, -12.9903) -> (-226.917, -12.6961)
  line L3993 (-226.917, -12.6961) -> (-227.0181, -12.2636)
  line L3994 (-227.0181, -12.2636) -> (-227.0786, -11.8246)
  line L3995 (-227.0786, -11.8246) -> (-227.0984, -11.3819)
  line L3996 (-227.0984, -11.3819) -> (-227.0771, -10.9382)
  line L3997 (-227.0928, 19.1125) -> (-227.0729, 19.52)
  line L3998 (-227.0729, 19.52) -> (-227.0211, 19.9239)
  line L3999 (-227.0211, 19.9239) -> (-226.9378, 20.3226)
  line L4000 (-226.9378, 20.3226) -> (-226.8232, 20.7141)
  line L4001 (-226.8232, 20.7141) -> (-226.6829, 21.0373)
  line L4002 (-226.6829, 21.0373) -> (-226.5146, 21.3469)
  line L4003 (-226.5146, 21.3469) -> (-226.3402, 21.5786)
  line L4004 (-226.3402, 21.5786) -> (-226.1357, 21.7844)
  line L4005 (-226.1357, 21.7844) -> (-225.7718, 22.0143)
  line L4006 (-225.7718, 22.0143) -> (-225.3783, 22.1819)
  line L4007 (-225.3783, 22.1819) -> (-224.9632, 22.2845)
  line L4008 (-224.9632, 22.2845) -> (-224.5342, 22.3196)
  line L4009 (-224.5342, 22.3196) -> (-224.2257, 22.3327)
  line L4010 (-224.2257, 22.3327) -> (-223.917, 22.3391)
  line L4011 (-223.917, 22.3391) -> (-221.1045, 22.3391)
  line L4012 (-221.1045, 22.3391) -> (-220.1958, 22.3515)
  line L4013 (-220.1958, 22.3515) -> (-219.2881, 22.3938)
  line L4014 (-219.2881, 22.3938) -> (-218.9031, 22.4384)
  line L4015 (-218.9031, 22.4384) -> (-218.5269, 22.5263)
  line L4016 (-218.5269, 22.5263) -> (-218.1631, 22.6563)
  line L4017 (-218.1631, 22.6563) -> (-217.8154, 22.8274)
  line L4018 (-217.8154, 22.8274) -> (-217.8154, 21.218)
  line L4019 (-217.8154, 21.218) -> (-218.0846, 21.1044)
  line L4020 (-218.0846, 21.1044) -> (-218.3623, 21.0154)
  line L4021 (-218.3623, 21.0154) -> (-218.6468, 20.9516)
  line L4022 (-218.6468, 20.9516) -> (-218.9365, 20.9133)
  line L4023 (-218.9365, 20.9133) -> (-218.6098, 20.5054)
  line L4024 (-218.6098, 20.5054) -> (-218.3154, 20.0735)
  line L4025 (-218.3154, 20.0735) -> (-218.092, 19.6813)
  line L4026 (-218.092, 19.6813) -> (-217.9092, 19.2688)
  line L4027 (-217.9092, 19.2688) -> (-217.7175, 18.6034)
  line L4028 (-217.7175, 18.6034) -> (-217.6205, 17.9212)
  line L4029 (-217.6205, 17.9212) -> (-217.6191, 17.2321)
  line L4030 (-217.6191, 17.2321) -> (-217.7139, 16.5461)
  line L4031 (-217.7139, 16.5461) -> (-217.7873, 16.2642)
  line L4032 (-217.7873, 16.2642) -> (-217.8886, 15.9917)
  line L4033 (-217.8886, 15.9917) -> (-218.0167, 15.7309)
  line L4034 (-218.0167, 15.7309) -> (-218.1709, 15.4836)
  line L4035 (-218.1709, 15.4836) -> (-218.36, 15.2516)
  line L4036 (-218.36, 15.2516) -> (-218.5737, 15.0467)
  line L4037 (-218.5737, 15.0467) -> (-218.8089, 14.8703)
  line L4038 (-218.8089, 14.8703) -> (-219.0628, 14.7239)
  line L4039 (-219.0628, 14.7239) -> (-219.3323, 14.6091)
  line L4040 (-219.3323, 14.6091) -> (-219.6147, 14.5272)
  line L4041 (-219.6147, 14.5272) -> (-219.9069, 14.4797)
  line L4042 (-219.9069, 14.4797) -> (-220.206, 14.468)
  line L4043 (-220.206, 14.468) -> (-220.5565, 14.4913)
  line L4044 (-220.5565, 14.4913) -> (-220.8957, 14.5611)
  line L4045 (-220.8957, 14.5611) -> (-221.2196, 14.6749)
  line L4046 (-221.2196, 14.6749) -> (-221.5242, 14.8304)
  line L4047 (-221.5242, 14.8304) -> (-221.8054, 15.025)
  line L4048 (-221.8054, 15.025) -> (-222.0591, 15.2563)
  line L4049 (-222.0591, 15.2563) -> (-222.2812, 15.522)
  line L4050 (-222.2812, 15.522) -> (-222.4678, 15.8196)
  line L4051 (-222.4678, 15.8196) -> (-222.6321, 16.1581)
  line L4052 (-222.6321, 16.1581) -> (-222.7648, 16.5094)
  line L4053 (-222.7648, 16.5094) -> (-222.8652, 16.8712)
  line L4054 (-222.8652, 16.8712) -> (-222.9326, 17.2414)
  line L4055 (-222.9326, 17.2414) -> (-223.0714, 18.2715)
  line L4056 (-223.0714, 18.2715) -> (-223.2217, 19.3)
  line L4057 (-223.2217, 19.3) -> (-223.3677, 20.0493)
  line L4058 (-223.3677, 20.0493) -> (-223.5732, 20.7844)
  line L4059 (-223.5732, 20.7844) -> (-224.0905, 20.7877)
  line L4060 (-224.0905, 20.7877) -> (-224.6045, 20.7297)
  line L4061 (-224.6045, 20.7297) -> (-224.9149, 20.6288)
  line L4062 (-224.9149, 20.6288) -> (-225.1943, 20.4602)
  line L4063 (-225.1943, 20.4602) -> (-225.3619, 20.2792)
  line L4064 (-225.3619, 20.2792) -> (-225.5017, 20.0774)
  line L4065 (-225.5017, 20.0774) -> (-225.6118, 19.8581)
  line L4066 (-225.6118, 19.8581) -> (-225.6904, 19.6243)
  line L4067 (-225.6904, 19.6243) -> (-225.7623, 19.3088)
  line L4068 (-225.7623, 19.3088) -> (-225.8072, 18.9889)
  line L4069 (-225.8072, 18.9889) -> (-225.8249, 18.6664)
  line L4070 (-225.8249, 18.6664) -> (-225.8154, 18.343)
  line L4071 (-225.8154, 18.343) -> (-225.7962, 18.0314)
  line L4072 (-225.7962, 18.0314) -> (-225.7418, 17.7251)
  line L4073 (-225.7418, 17.7251) -> (-225.6529, 17.4269)
  line L4074 (-225.6529, 17.4269) -> (-225.5303, 17.1399)
  line L4075 (-225.5303, 17.1399) -> (-225.4077, 16.9633)
  line L4076 (-225.4077, 16.9633) -> (-225.2632, 16.8055)
  line L4077 (-225.2632, 16.8055) -> (-225.099, 16.6683)
  line L4078 (-225.099, 16.6683) -> (-224.917, 16.5539)
  line L4079 (-224.917, 16.5539) -> (-224.5173, 16.3685)
  line L4080 (-224.5173, 16.3685) -> (-224.0967, 16.2375)
  line L4081 (-224.0967, 16.2375) -> (-224.2998, 14.7336)
  line L4082 (-224.2998, 14.7336) -> (-224.7438, 14.8494)
  line L4083 (-224.7438, 14.8494) -> (-225.1748, 15.0071)
  line L4084 (-225.1748, 15.0071) -> (-225.542, 15.1907)
  line L4085 (-225.542, 15.1907) -> (-225.8623, 15.4094)
  line L4086 (-225.8623, 15.4094) -> (-226.1218, 15.6551)
  line L4087 (-226.1218, 15.6551) -> (-226.3479, 15.9299)
  line L4088 (-226.3479, 15.9299) -> (-226.5382, 16.2307)
  line L4089 (-226.5382, 16.2307) -> (-226.6904, 16.5539)
  line L4090 (-226.6904, 16.5539) -> (-226.7764, 16.7688)
  line L4091 (-226.7764, 16.7688) -> (-226.9162, 17.2422)
  line L4092 (-226.9162, 17.2422) -> (-227.0146, 17.7258)
  line L4093 (-227.0146, 17.7258) -> (-227.0841, 18.4175)
  line L4094 (-227.0841, 18.4175) -> (-227.0928, 19.1125)
  line L4095 (-227.0849, 4.4914) -> (-227.0447, 4.8948)
  line L4096 (-227.0447, 4.8948) -> (-226.9623, 5.2905)
  line L4097 (-226.9623, 5.2905) -> (-226.8388, 5.6754)
  line L4098 (-226.8388, 5.6754) -> (-226.6748, 6.0461)
  line L4099 (-226.6748, 6.0461) -> (-226.3913, 6.4912)
  line L4100 (-226.3913, 6.4912) -> (-226.0401, 6.8803)
  line L4101 (-226.0401, 6.8803) -> (-225.6293, 7.2058)
  line L4102 (-225.6293, 7.2058) -> (-225.167, 7.4602)
  line L4103 (-225.167, 7.4602) -> (-224.7055, 7.6364)
  line L4104 (-224.7055, 7.6364) -> (-224.2256, 7.7532)
  line L4105 (-224.2256, 7.7532) -> (-223.9951, 6.2571)
  line L4106 (-223.9951, 6.2571) -> (-224.2495, 6.193)
  line L4107 (-224.2495, 6.193) -> (-224.4962, 6.1054)
  line L4108 (-224.4962, 6.1054) -> (-224.7335, 5.995)
  line L4109 (-224.7335, 5.995) -> (-224.9599, 5.8625)
  line L4110 (-224.9599, 5.8625) -> (-225.159, 5.7124)
  line L4111 (-225.159, 5.7124) -> (-225.335, 5.5401)
  line L4112 (-225.335, 5.5401) -> (-225.4867, 5.3483)
  line L4113 (-225.4867, 5.3483) -> (-225.6127, 5.1397)
  line L4114 (-225.6127, 5.1397) -> (-225.7114, 4.917)
  line L4115 (-225.7114, 4.917) -> (-225.7817, 4.6829)
  line L4116 (-225.7817, 4.6829) -> (-225.822, 4.4398)
  line L4117 (-225.822, 4.4398) -> (-225.831, 4.1907)
  line L4118 (-225.831, 4.1907) -> (-225.8085, 3.7912)
  line L4119 (-225.8085, 3.7912) -> (-225.7213, 3.4036)
  line L4120 (-225.7213, 3.4036) -> (-225.5717, 3.0354)
  line L4121 (-225.5717, 3.0354) -> (-225.3623, 2.6946)
  line L4122 (-225.3623, 2.6946) -> (-225.129, 2.4257)
  line L4123 (-225.129, 2.4257) -> (-224.8607, 2.1946)
  line L4124 (-224.8607, 2.1946) -> (-224.562, 2.0044)
  line L4125 (-224.562, 2.0044) -> (-224.2373, 1.8586)
  line L4126 (-224.2373, 1.8586) -> (-223.8854, 1.7502)
  line L4127 (-223.8854, 1.7502) -> (-223.5269, 1.6689)
  line L4128 (-223.5269, 1.6689) -> (-223.1632, 1.6151)
  line L4129 (-223.1632, 1.6151) -> (-222.7959, 1.5891)
  line L4130 (-222.7959, 1.5891) -> (-222.3785, 1.5741)
  line L4131 (-222.3785, 1.5741) -> (-221.9613, 1.5835)
  line L4132 (-221.9613, 1.5835) -> (-221.5454, 1.6172)
  line L4133 (-221.5454, 1.6172) -> (-221.1318, 1.675)
  line L4134 (-221.1318, 1.675) -> (-220.8155, 1.7411)
  line L4135 (-220.8155, 1.7411) -> (-220.5076, 1.8365)
  line L4136 (-220.5076, 1.8365) -> (-220.21, 1.9606)
  line L4137 (-220.21, 1.9606) -> (-219.9248, 2.1125)
  line L4138 (-219.9248, 2.1125) -> (-219.6174, 2.3519)
  line L4139 (-219.6174, 2.3519) -> (-219.356, 2.6371)
  line L4140 (-219.356, 2.6371) -> (-219.1456, 2.9619)
  line L4141 (-219.1456, 2.9619) -> (-218.9912, 3.3196)
  line L4142 (-218.9912, 3.3196) -> (-218.909, 3.6706)
  line L4143 (-218.909, 3.6706) -> (-218.875, 4.0279)
  line L4144 (-218.875, 4.0279) -> (-218.8894, 4.3864)
  line L4145 (-218.8894, 4.3864) -> (-218.9521, 4.7414)
  line L4146 (-218.9521, 4.7414) -> (-219.0247, 4.9672)
  line L4147 (-219.0247, 4.9672) -> (-219.1219, 5.1809)
  line L4148 (-219.1219, 5.1809) -> (-219.2421, 5.3808)
  line L4149 (-219.2421, 5.3808) -> (-219.3838, 5.5652)
  line L4150 (-219.3838, 5.5652) -> (-219.5455, 5.7324)
  line L4151 (-219.5455, 5.7324) -> (-219.7258, 5.8805)
  line L4152 (-219.7258, 5.8805) -> (-219.923, 6.0078)
  line L4153 (-219.923, 6.0078) -> (-220.1357, 6.1125)
  line L4154 (-220.1357, 6.1125) -> (-220.6281, 6.2845)
  line L4155 (-220.6281, 6.2845) -> (-221.1396, 6.386)
  line L4156 (-221.1396, 6.386) -> (-220.9443, 7.8977)
  line L4157 (-220.9443, 7.8977) -> (-220.5835, 7.8302)
  line L4158 (-220.5835, 7.8302) -> (-220.2296, 7.7344)
  line L4159 (-220.2296, 7.7344) -> (-219.8845, 7.6109)
  line L4160 (-219.8845, 7.6109) -> (-219.5498, 7.4602)
  line L4161 (-219.5498, 7.4602) -> (-219.1853, 7.2436)
  line L4162 (-219.1853, 7.2436) -> (-218.8526, 6.988)
  line L4163 (-218.8526, 6.988) -> (-218.5542, 6.697)
  line L4164 (-218.5542, 6.697) -> (-218.2928, 6.3741)
  line L4165 (-218.2928, 6.3741) -> (-218.0708, 6.0229)
  line L4166 (-218.0708, 6.0229) -> (-217.8908, 5.647)
  line L4167 (-217.8908, 5.647) -> (-217.7553, 5.2499)
  line L4168 (-217.7553, 5.2499) -> (-217.667, 4.8352)
  line L4169 (-217.667, 4.8352) -> (-217.6146, 4.3308)
  line L4170 (-217.6146, 4.3308) -> (-217.6162, 3.8252)
  line L4171 (-217.6162, 3.8252) -> (-217.6715, 3.3226)
  line L4172 (-217.6715, 3.3226) -> (-217.7803, 2.8274)
  line L4173 (-217.7803, 2.8274) -> (-217.9519, 2.3513)
  line L4174 (-217.9519, 2.3513) -> (-218.1861, 1.9053)
  line L4175 (-218.1861, 1.9053) -> (-218.4791, 1.4956)
  line L4176 (-218.4791, 1.4956) -> (-218.8271, 1.1282)
  line L4177 (-218.8271, 1.1282) -> (-219.1474, 0.8625)
  line L4178 (-219.1474, 0.8625) -> (-219.5071, 0.6297)
  line L4179 (-219.5071, 0.6297) -> (-219.8896, 0.4368)
  line L4180 (-219.8896, 0.4368) -> (-220.3076, 0.2766)
  line L4181 (-220.3076, 0.2766) -> (-220.6663, 0.1776)
  line L4182 (-220.6663, 0.1776) -> (-221.03, 0.1008)
  line L4183 (-221.03, 0.1008) -> (-221.3978, 0.0465)
  line L4184 (-221.3978, 0.0465) -> (-221.7685, 0.0149)
  line L4185 (-221.7685, 0.0149) -> (-222.2526, -0.0047)
  line L4186 (-222.2526, -0.0047) -> (-222.7365, 0.0058)
  line L4187 (-222.7365, 0.0058) -> (-223.2189, 0.0462)
  line L4188 (-223.2189, 0.0462) -> (-223.6982, 0.1164)
  line L4189 (-223.6982, 0.1164) -> (-224.1468, 0.2168)
  line L4190 (-224.1468, 0.2168) -> (-224.5833, 0.3577)
  line L4191 (-224.5833, 0.3577) -> (-225.005, 0.5381)
  line L4192 (-225.005, 0.5381) -> (-225.4092, 0.7571)
  line L4193 (-225.4092, 0.7571) -> (-225.8538, 1.0979)
  line L4194 (-225.8538, 1.0979) -> (-226.2357, 1.503)
  line L4195 (-226.2357, 1.503) -> (-226.5481, 1.9638)
  line L4196 (-226.5481, 1.9638) -> (-226.7842, 2.4719)
  line L4197 (-226.7842, 2.4719) -> (-226.9445, 2.9617)
  line L4198 (-226.9445, 2.9617) -> (-227.0486, 3.4647)
  line L4199 (-227.0486, 3.4647) -> (-227.0956, 3.9762)
  line L4200 (-227.0956, 3.9762) -> (-227.0849, 4.4914)
  line L4201 (-227.0771, -29.3445) -> (-227.0391, -29.0266)
  line L4202 (-227.0391, -29.0266) -> (-226.9781, -28.7128)
  line L4203 (-226.9781, -28.7128) -> (-226.8943, -28.4043)
  line L4204 (-226.8943, -28.4043) -> (-226.7881, -28.1023)
  line L4205 (-226.7881, -28.1023) -> (-226.6626, -27.8208)
  line L4206 (-226.6626, -27.8208) -> (-226.5148, -27.551)
  line L4207 (-226.5148, -27.551) -> (-226.3454, -27.2941)
  line L4208 (-226.3454, -27.2941) -> (-226.1553, -27.0515)
  line L4209 (-226.1553, -27.0515) -> (-225.8701, -26.7429)
  line L4210 (-225.8701, -26.7429) -> (-225.547, -26.4665)
  line L4211 (-225.547, -26.4665) -> (-225.1982, -26.2234)
  line L4212 (-225.1982, -26.2234) -> (-224.9067, -26.0633)
  line L4213 (-224.9067, -26.0633) -> (-224.6042, -25.9263)
  line L4214 (-224.6042, -25.9263) -> (-224.292, -25.8128)
  line L4215 (-224.292, -25.8128) -> (-223.9717, -25.7234)
  line L4216 (-223.9717, -25.7234) -> (-223.6028, -25.6486)
  line L4217 (-223.6028, -25.6486) -> (-223.2305, -25.5957)
  line L4218 (-223.2305, -25.5957) -> (-222.8557, -25.5646)
  line L4219 (-222.8557, -25.5646) -> (-222.4795, -25.5554)
  line L4220 (-222.4795, -25.5554) -> (-222.0018, -25.5624)
  line L4221 (-222.0018, -25.5624) -> (-221.526, -25.5987)
  line L4222 (-221.526, -25.5987) -> (-221.0532, -25.6642)
  line L4223 (-221.0532, -25.6642) -> (-220.5849, -25.7586)
  line L4224 (-220.5849, -25.7586) -> (-220.1711, -25.884)
  line L4225 (-220.1711, -25.884) -> (-219.778, -26.054)
  line L4226 (-219.778, -26.054) -> (-219.409, -26.266)
  line L4227 (-219.409, -26.266) -> (-219.067, -26.5174)
  line L4228 (-219.067, -26.5174) -> (-218.7554, -26.8055)
  line L4229 (-218.7554, -26.8055) -> (-218.4772, -27.1278)
  line L4230 (-218.4772, -27.1278) -> (-218.2358, -27.4815)
  line L4231 (-218.2358, -27.4815) -> (-218.0342, -27.864)
  line L4232 (-218.0342, -27.864) -> (-217.8472, -28.3283)
  line L4233 (-217.8472, -28.3283) -> (-217.7133, -28.809)
  line L4234 (-217.7133, -28.809) -> (-217.6333, -29.3016)
  line L4235 (-217.6333, -29.3016) -> (-217.6084, -29.8015)
  line L4236 (-217.6084, -29.8015) -> (-217.6182, -30.1373)
  line L4237 (-217.6182, -30.1373) -> (-217.6502, -30.4713)
  line L4238 (-217.6502, -30.4713) -> (-217.7043, -30.8025)
  line L4239 (-217.7043, -30.8025) -> (-217.7803, -31.1296)
  line L4240 (-217.7803, -31.1296) -> (-217.8772, -31.4239)
  line L4241 (-217.8772, -31.4239) -> (-217.9959, -31.7096)
  line L4242 (-217.9959, -31.7096) -> (-218.1356, -31.9856)
  line L4243 (-218.1356, -31.9856) -> (-218.2959, -32.2507)
  line L4244 (-218.2959, -32.2507) -> (-218.5474, -32.5807)
  line L4245 (-218.5474, -32.5807) -> (-218.831, -32.8836)
  line L4246 (-218.831, -32.8836) -> (-219.1568, -33.1581)
  line L4247 (-219.1568, -33.1581) -> (-219.5107, -33.3953)
  line L4248 (-219.5107, -33.3953) -> (-219.907, -33.601)
  line L4249 (-219.907, -33.601) -> (-220.3232, -33.7625)
  line L4250 (-220.3232, -33.7625) -> (-220.6842, -33.8668)
  line L4251 (-220.6842, -33.8668) -> (-221.0507, -33.9479)
  line L4252 (-221.0507, -33.9479) -> (-221.4217, -34.0056)
  line L4253 (-221.4217, -34.0056) -> (-221.7959, -34.0398)
  line L4254 (-221.7959, -34.0398) -> (-222.3799, -34.0554)
  line L4255 (-222.3799, -34.0554) -> (-222.9639, -34.0359)
  line L4256 (-222.9639, -34.0359) -> (-223.5303, -33.9695)
  line L4257 (-223.5303, -33.9695) -> (-224.0576, -33.8601)
  line L4258 (-224.0576, -33.8601) -> (-224.5459, -33.7078)
  line L4259 (-224.5459, -33.7078) -> (-224.9912, -33.5086)
  line L4260 (-224.9912, -33.5086) -> (-225.3974, -33.2703)
  line L4261 (-225.3974, -33.2703) -> (-225.7646, -32.9851)
  line L4262 (-225.7646, -32.9851) -> (-226.0849, -32.657)
  line L4263 (-226.0849, -32.657) -> (-226.4287, -32.1996)
  line L4264 (-226.4287, -32.1996) -> (-226.7033, -31.7008)
  line L4265 (-226.7033, -31.7008) -> (-226.905, -31.1684)
  line L4266 (-226.905, -31.1684) -> (-227.0303, -30.6101)
  line L4267 (-227.0303, -30.6101) -> (-227.0719, -30.2953)
  line L4268 (-227.0719, -30.2953) -> (-227.0936, -29.9788)
  line L4269 (-227.0936, -29.9788) -> (-227.0954, -29.6615)
  line L4270 (-227.0954, -29.6615) -> (-227.0771, -29.3445)
  line L4271 (-226.8896, 31.675) -> (-226.8896, 33.2219)
  line L4272 (-226.8896, 33.2219) -> (-225.6943, 33.2219)
  line L4273 (-225.6943, 33.2219) -> (-225.6943, 31.675)
  line L4274 (-225.6943, 31.675) -> (-220.3857, 31.675)
  line L4275 (-220.3857, 31.675) -> (-220.0235, 31.684)
  line L4276 (-220.0235, 31.684) -> (-219.6631, 31.7219)
  line L4277 (-219.6631, 31.7219) -> (-219.4812, 31.7901)
  line L4278 (-219.4812, 31.7901) -> (-219.3307, 31.9062)
  line L4279 (-219.3307, 31.9062) -> (-219.2204, 32.061)
  line L4280 (-219.2204, 32.061) -> (-219.1592, 32.2454)
  line L4281 (-219.1592, 32.2454) -> (-219.1384, 32.4899)
  line L4282 (-219.1384, 32.4899) -> (-219.1368, 32.7348)
  line L4283 (-219.1368, 32.7348) -> (-219.1541, 32.9792)
  line L4284 (-219.1541, 32.9792) -> (-219.1904, 33.2219)
  line L4285 (-219.1904, 33.2219) -> (-217.831, 33.4446)
  line L4286 (-217.831, 33.4446) -> (-217.7441, 32.9723)
  line L4287 (-217.7441, 32.9723) -> (-217.7033, 32.4949)